Autodesk Inventor part; units mm, degrees
(part 2 of 4)
sketch "スケッチ16" plane through (0, 0, 0) normal (0, 0, 1) x (1, 0, 0)
  line L0 (45.3386, -92.477) -> (54.3014, -95.75) projected
  line L1 (54.3014, -95.75) -> (66.3014, -95.75) projected
  line L2 (66.3014, -95.75) -> (66.3014, -95.339) projected
  arc A0 (74.7167, -80.1031) -> (66.3014, -95.339) centre (84.3014, -95.339) ccw projected
  line L3 (74.7167, -80.1031) -> (119.8722, -51.6966) projected
  arc A1 (119.8722, -51.6966) -> (121.0577, -50.8686) centre (111.885, -39) ccw projected
  line L4 (121.0577, -50.8686) -> (127.6513, -45.7727) projected
  line L5 (127.6513, -45.7727) -> (126.8081, -37.4821) projected
  arc A2 (126.8081, -37.4821) -> (124.1514, -30.3665) centre (111.885, -39) ccw projected
  line L6 (124.1514, -30.3665) -> (104.8897, -3) projected
  line L7 (104.8897, -3) -> (101.8897, -3) projected
  arc A3 (99.8897, -3) -> (101.8897, -3) centre (100.8897, -3) ccw projected
  line L8 (99.8897, -3) -> (99.8897, 0) projected
  line L9 (99.8897, 0) -> (84.8897, 0) projected
  line L10 (84.8897, 0) -> (84.8897, -3) projected
  arc A4 (82.8897, -3) -> (84.8897, -3) centre (83.8897, -3) ccw projected
  line L11 (82.8897, -3) -> (71.4443, -3) projected
  arc A5 (69.4443, -3) -> (71.4443, -3) centre (70.4443, -3) ccw projected
  line L12 (69.4443, -3) -> (69.4443, 0) projected
  line L13 (69.4443, 0) -> (54.4443, 0) projected
  line L14 (54.4443, 0) -> (54.4443, -3) projected
  arc A6 (52.4443, -3) -> (54.4443, -3) centre (53.4443, -3) ccw projected
  line L15 (52.4443, -3) -> (49.4443, -3) projected
  line L16 (49.4443, -3) -> (49.4443, -6) projected
  line L17 (49.4443, -6) -> (53.9457, -9.7931) projected
  arc A7 (54.3014, -10.5578) -> (53.9457, -9.7931) centre (53.3014, -10.5578) ccw projected
  line L18 (54.3014, -10.5578) -> (54.3014, -82.75) projected
  arc A8 (53.3014, -83.75) -> (54.3014, -82.75) centre (53.3014, -82.75) ccw projected
  line L19 (53.3014, -83.75) -> (46.8822, -83.75) projected
  arc A9 (46.8822, -83.75) -> (45.3386, -92.477) centre (46.8822, -88.25) ccw projected
  circle A10 centre (111.885, -39) radius 1.5 projected
  arc A11 (89.8897, -3) -> (87.8897, -3) centre (88.8897, -3) ccw projected
  line L20 (89.8897, -3) -> (94.8897, -3) projected
  arc A12 (96.8897, -3) -> (94.8897, -3) centre (95.8897, -3) ccw projected
  line L21 (96.8897, -3) -> (96.8897, -6) projected
  arc A13 (94.8897, -6) -> (96.8897, -6) centre (95.8897, -6) ccw projected
  line L22 (94.8897, -6) -> (89.8897, -6) projected
  arc A14 (87.8897, -6) -> (89.8897, -6) centre (88.8897, -6) ccw projected
  line L23 (87.8897, -6) -> (87.8897, -3) projected
  line L24 (57.4443, -6) -> (57.4443, -3) projected
  arc A15 (59.4443, -3) -> (57.4443, -3) centre (58.4443, -3) ccw projected
  line L25 (59.4443, -3) -> (64.4443, -3) projected
  arc A16 (66.4443, -3) -> (64.4443, -3) centre (65.4443, -3) ccw projected
  line L26 (66.4443, -3) -> (66.4443, -6) projected
  arc A17 (64.4443, -6) -> (66.4443, -6) centre (65.4443, -6) ccw projected
  line L27 (64.4443, -6) -> (59.4443, -6) projected
  arc A18 (57.4443, -6) -> (59.4443, -6) centre (58.4443, -6) ccw projected
  circle A19 centre (46.8822, -88.25) radius 1.5 projected
  circle A20 centre (47.8869, -88.25) radius 1.5
  line L28 (46.177, -92.4125) -> (54.3014, -95.75)
  line L29 (54.3014, -95.75) -> (66.3014, -95.75)
  line L30 (66.3014, -95.75) -> (66.3014, -95.339)
  arc A21 (74.7167, -80.1031) -> (66.3014, -95.339) centre (84.3014, -95.339) ccw
  line L31 (74.7167, -80.1031) -> (119.8722, -51.6966)
  arc A22 (119.8722, -51.6966) -> (121.0577, -50.8686) centre (111.885, -39) ccw
  line L32 (121.0577, -50.8686) -> (127.6513, -45.7727)
  line L33 (127.6513, -45.7727) -> (119.127, -45.896)
  arc A23 (104.885, -31.8586) -> (119.127, -45.896) centre (111.885, -39) ccw
  line L34 (104.885, -31.8586) -> (104.885, -3)
  line L35 (104.885, -3) -> (101.8897, -3)
  arc A24 (99.8897, -3) -> (101.8897, -3) centre (100.8897, -3) ccw
  line L36 (99.8897, -3) -> (96.8897, -3)
  line L37 (96.8897, -3) -> (96.8897, -6)
  arc A25 (94.8897, -6) -> (96.8897, -6) centre (95.8897, -6) ccw
  line L38 (94.8897, -6) -> (89.8897, -6)
  arc A26 (87.8897, -6) -> (89.8897, -6) centre (88.8897, -6) ccw
  line L39 (87.8897, -6) -> (87.8897, -3)
  line L40 (87.8897, -3) -> (84.8897, -3)
  arc A27 (82.8897, -3) -> (84.8897, -3) centre (83.8897, -3) ccw
  line L41 (82.8897, -3) -> (71.4443, -3)
  arc A28 (69.4443, -3) -> (71.4443, -3) centre (70.4443, -3) ccw
  line L42 (69.4443, -3) -> (66.4443, -3)
  line L43 (66.4443, -3) -> (66.4443, -6)
  arc A29 (64.4443, -6) -> (66.4443, -6) centre (65.4443, -6) ccw
  line L44 (64.4443, -6) -> (59.4443, -6)
  arc A30 (57.4443, -6) -> (59.4443, -6) centre (58.4443, -6) ccw
  line L45 (57.4443, -6) -> (57.4443, -3)
  line L46 (57.4443, -3) -> (54.4443, -3)
  arc A31 (52.4443, -3) -> (54.4443, -3) centre (53.4443, -3) ccw
  line L47 (52.4443, -3) -> (49.4443, -3)
  line L48 (49.4443, -3) -> (49.4443, -6)
  line L49 (49.4443, -6) -> (53.9457, -9.7931)
  arc A32 (54.3014, -10.5578) -> (53.9457, -9.7931) centre (53.3014, -10.5578) ccw
  line L50 (54.3014, -10.5578) -> (54.3014, -82.75)
  arc A33 (53.3014, -83.75) -> (54.3014, -82.75) centre (53.3014, -82.75) ccw
  line L51 (53.3014, -83.75) -> (47.8869, -83.75)
  arc A34 (47.8869, -83.75) -> (46.177, -92.4125) centre (47.8869, -88.25) ccw
  point P0 (0, 0)
  point P1 (0, 0)
  point P2 (47.885, -83.75)
  constraints: 48 end point, 28 point on circle, 21 horizontal, 19 vertical, 15 centre point, 168 other
extrude "押し出し19" add sketch "スケッチ16" against normal blind 5 contours A19 A20 | A20 A19 picked at (47.067, -88.3717) picked at (46.0813, -88.0099)
extrude "押し出し20" cut sketch "スケッチ16" against normal blind 10 contours A9 L19 A34 L28 L0
hole "穴2" at (47.8869, -88.25, 0) direction (0, 0, -1) diameter 3 depth 12 tip angle 118
sketch "スケッチ17" plane through (0, 0, -5) normal (0, 0, -1) x (-1, 0, 0)
  circle A0 centre (-47.8869, -88.25) radius 1.5 projected
  arc A1 (-46.177, -92.4125) -> (-47.885, -83.75) centre (-47.8869, -88.25) ccw projected
  line L0 (-47.885, -83.75) -> (-53.3014, -83.75) projected
  arc A2 (-54.3014, -82.75) -> (-53.3014, -83.75) centre (-53.3014, -82.75) ccw projected
  line L1 (-54.3014, -82.75) -> (-54.3014, -10.5578) projected
  arc A3 (-53.9457, -9.7931) -> (-54.3014, -10.5578) centre (-53.3014, -10.5578) ccw projected
  line L2 (-53.9457, -9.7931) -> (-49.4443, -6) projected
  line L3 (-49.4443, -6) -> (-49.4443, -3) projected
  line L4 (-49.4443, -3) -> (-52.4443, -3) projected
  arc A4 (-54.4443, -3) -> (-52.4443, -3) centre (-53.4443, -3) ccw projected
  line L5 (-54.4443, -3) -> (-57.4443, -3) projected
  line L6 (-57.4443, -3) -> (-57.4443, -6) projected
  arc A5 (-59.4443, -6) -> (-57.4443, -6) centre (-58.4443, -6) ccw projected
  line L7 (-59.4443, -6) -> (-64.4443, -6) projected
  arc A6 (-66.4443, -6) -> (-64.4443, -6) centre (-65.4443, -6) ccw projected
  line L8 (-66.4443, -6) -> (-66.4443, -3) projected
  line L9 (-66.4443, -3) -> (-69.4443, -3) projected
  arc A7 (-71.4443, -3) -> (-69.4443, -3) centre (-70.4443, -3) ccw projected
  line L10 (-71.4443, -3) -> (-82.8897, -3) projected
  arc A8 (-84.8897, -3) -> (-82.8897, -3) centre (-83.8897, -3) ccw projected
  line L11 (-84.8897, -3) -> (-87.8897, -3) projected
  line L12 (-87.8897, -3) -> (-87.8897, -6) projected
  arc A9 (-89.8897, -6) -> (-87.8897, -6) centre (-88.8897, -6) ccw projected
  line L13 (-89.8897, -6) -> (-94.8897, -6) projected
  arc A10 (-96.8897, -6) -> (-94.8897, -6) centre (-95.8897, -6) ccw projected
  line L14 (-96.8897, -6) -> (-96.8897, -3) projected
  line L15 (-96.8897, -3) -> (-99.8897, -3) projected
  arc A11 (-101.8897, -3) -> (-99.8897, -3) centre (-100.8897, -3) ccw projected
  line L16 (-101.8897, -3) -> (-104.885, -3) projected
  line L17 (-104.885, -3) -> (-104.885, -31.8586) projected
  arc A12 (-119.127, -45.896) -> (-104.885, -31.8586) centre (-111.885, -39) ccw projected
  line L18 (-119.127, -45.896) -> (-127.6513, -45.7727) projected
  line L19 (-127.6513, -45.7727) -> (-121.0577, -50.8686) projected
  arc A13 (-121.0577, -50.8686) -> (-119.8722, -51.6966) centre (-111.885, -39) ccw projected
  line L20 (-119.8722, -51.6966) -> (-74.7167, -80.1031) projected
  arc A14 (-66.3014, -95.339) -> (-74.7167, -80.1031) centre (-84.3014, -95.339) ccw projected
  line L21 (-66.3014, -95.339) -> (-66.3014, -95.75) projected
  line L22 (-66.3014, -95.75) -> (-54.3014, -95.75) projected
  line L23 (-54.3014, -95.75) -> (-46.177, -92.4125) projected
  line L24 (-71.5218, -75.0244) -> (-116.6774, -46.618)
  arc A15 (-117.3886, -46.1211) -> (-116.6774, -46.618) centre (-111.885, -39) ccw
  line L25 (-117.3886, -46.1211) -> (-127.8557, -38.0317)
  arc A16 (-127.8557, -38.0317) -> (-98.885, -29.6726) centre (-111.885, -39) ccw
  line L26 (-98.885, -29.6726) -> (-98.885, -12.3268)
  arc A17 (-98.885, -12.3268) -> (-92.3897, -12.0622) centre (-95.8897, -6) ccw
  arc A18 (-92.3897, -12.0622) -> (-81.8897, -6) centre (-88.8897, -6) ccw
  line L27 (-81.8897, -6) -> (-81.8897, 3.7082)
  arc A19 (-81.8897, 3.7082) -> (-80.2841, -9) centre (-83.8897, -3) ccw
  line L28 (-80.2841, -9) -> (-74.0499, -9)
  arc A20 (-74.0499, -9) -> (-72.4443, 3.7082) centre (-70.4443, -3) ccw
  line L29 (-72.4443, 3.7082) -> (-72.4443, -6)
  arc A21 (-72.4443, -6) -> (-61.9443, 0.0622) centre (-65.4443, -6) ccw
  arc A22 (-61.9443, 0.0622) -> (-60.3014, -12.7492) centre (-58.4443, -6) ccw
  line L30 (-60.3014, -12.7492) -> (-60.3014, -82.75)
  arc A23 (-60.3014, -82.75) -> (-54.9853, -89.5444) centre (-53.3014, -82.75) ccw
  line L31 (-54.9853, -89.5444) -> (-55.4858, -89.75)
  line L32 (-55.4858, -89.75) -> (-60.9612, -89.75)
  arc A24 (-60.9612, -89.75) -> (-71.5218, -75.0244) centre (-84.3014, -95.339) ccw
  arc A25 (-58.5929, -89.75) -> (-57.9314, -88) centre (-58.5929, -88.75) ccw
  point P0 (0, 0)
  point P1 (-105.48, -53.662)
  point P2 (-61.9443, -12.0622)
  point P3 (-71.2186, -9.9571)
  point P4 (-83.1155, -9.9571)
  dimension "d164" = 6
  dimension "d166" = 2
  constraints: 23 point on circle, 18 end point, 11 centre point, 2 tangent, 1 point on line, 18 other
  measures "d164" distance between parallel lines of L20 L24
  measures "d166" diameter of A25
extrude "押し出し21" cut sketch "スケッチ17" against normal blind 4 contours A16 L26 A17 A18 A19 L28 A20 A21 A22 L30 A23 A25 L32 A24 L24
fillet "フィレット3" radius 1 11 edges at (60.9612, -89.75, -3) (105.48, -53.662, -3) (98.885, -29.6726, -3) (98.885, -12.3268, -3) (92.3897, -12.0622, -3) (83.1155, -9.9571, -3) (80.2841, -9, -3) (74.0499, -9, -3) (71.2186, -9.9571, -3) (61.9443, -12.0622, -3) (60.3014, -12.7492, -3)
sketch "スケッチ18" plane through (0, 0, -5) normal (0, 0, -1) x (-1, 0, 0)
  arc A0 (-82.7234, -9.9022) -> (-80.5008, -9.125) centre (-83.8897, -3) ccw projected
  arc A1 (-80.0167, -9) -> (-80.5008, -9.125) centre (-80.0167, -10) ccw projected
  line L0 (-80.0167, -9) -> (-74.3173, -9) projected
  arc A2 (-73.8332, -9.125) -> (-74.3173, -9) centre (-74.3173, -10) ccw projected
  arc A3 (-73.8332, -9.125) -> (-71.6106, -9.9022) centre (-70.4443, -3) ccw projected
  arc A4 (-70.9856, -10.2772) -> (-71.6106, -9.9022) centre (-71.7772, -10.8882) ccw projected
  arc A5 (-70.9856, -10.2772) -> (-62.3818, -12.2945) centre (-65.4443, -6) ccw projected
  arc A6 (-61.5068, -12.2945) -> (-62.3818, -12.2945) centre (-61.9443, -13.1937) ccw projected
  arc A7 (-61.5068, -12.2945) -> (-60.9442, -12.5384) centre (-58.4443, -6) ccw projected
  arc A8 (-60.3014, -13.4724) -> (-60.9442, -12.5384) centre (-61.3014, -13.4724) ccw projected
  line L1 (-60.3014, -13.4724) -> (-60.3014, -82.75) projected
  arc A9 (-60.3014, -82.75) -> (-57.9314, -88) centre (-53.3014, -82.75) ccw projected
  arc A10 (-58.5929, -89.75) -> (-57.9314, -88) centre (-58.5929, -88.75) ccw projected
  line L2 (-58.5929, -89.75) -> (-60.1853, -89.75) projected
  arc A11 (-61.1499, -89.0136) -> (-60.1853, -89.75) centre (-60.1853, -88.75) ccw projected
  arc A12 (-61.1499, -89.0136) -> (-71.5218, -75.0244) centre (-84.3014, -95.339) ccw projected
  line L3 (-71.5218, -75.0244) -> (-103.9807, -54.6052) projected
  arc A13 (-103.9445, -52.8906) -> (-103.9807, -54.6052) centre (-103.4483, -53.7587) ccw projected
  arc A14 (-103.9445, -52.8906) -> (-98.7086, -29.9236) centre (-111.885, -39) ccw projected
  arc A15 (-98.885, -29.3564) -> (-98.7086, -29.9236) centre (-97.885, -29.3564) ccw projected
  line L4 (-98.885, -29.3564) -> (-98.885, -13.7472) projected
  arc A16 (-97.6356, -12.7788) -> (-98.885, -13.7472) centre (-97.885, -13.7472) ccw projected
  arc A17 (-97.6356, -12.7788) -> (-92.8272, -12.2945) centre (-95.8897, -6) ccw projected
  arc A18 (-91.9522, -12.2945) -> (-92.8272, -12.2945) centre (-92.3897, -13.1937) ccw projected
  arc A19 (-91.9522, -12.2945) -> (-83.3484, -10.2772) centre (-88.8897, -6) ccw projected
  arc A20 (-82.7234, -9.9022) -> (-83.3484, -10.2772) centre (-82.5568, -10.8882) ccw projected
  circle A21 centre (-47.8869, -88.25) radius 1.5 projected
  arc A22 (-46.177, -92.4125) -> (-47.885, -83.75) centre (-47.8869, -88.25) ccw projected
  line L5 (-47.885, -83.75) -> (-53.3014, -83.75) projected
  arc A23 (-54.3014, -82.75) -> (-53.3014, -83.75) centre (-53.3014, -82.75) ccw projected
  line L6 (-54.3014, -82.75) -> (-54.3014, -10.5578) projected
  arc A24 (-53.9457, -9.7931) -> (-54.3014, -10.5578) centre (-53.3014, -10.5578) ccw projected
  line L7 (-53.9457, -9.7931) -> (-49.4443, -6) projected
  line L8 (-49.4443, -6) -> (-49.4443, -3) projected
  line L9 (-49.4443, -3) -> (-52.4443, -3) projected
  arc A25 (-54.4443, -3) -> (-52.4443, -3) centre (-53.4443, -3) ccw projected
  line L10 (-54.4443, -3) -> (-57.4443, -3) projected
  line L11 (-57.4443, -3) -> (-57.4443, -6) projected
  arc A26 (-59.4443, -6) -> (-57.4443, -6) centre (-58.4443, -6) ccw projected
  line L12 (-59.4443, -6) -> (-64.4443, -6) projected
  arc A27 (-66.4443, -6) -> (-64.4443, -6) centre (-65.4443, -6) ccw projected
  line L13 (-66.4443, -6) -> (-66.4443, -3) projected
  line L14 (-66.4443, -3) -> (-69.4443, -3) projected
  arc A28 (-71.4443, -3) -> (-69.4443, -3) centre (-70.4443, -3) ccw projected
  line L15 (-71.4443, -3) -> (-82.8897, -3) projected
  arc A29 (-84.8897, -3) -> (-82.8897, -3) centre (-83.8897, -3) ccw projected
  line L16 (-84.8897, -3) -> (-87.8897, -3) projected
  line L17 (-87.8897, -3) -> (-87.8897, -6) projected
  arc A30 (-89.8897, -6) -> (-87.8897, -6) centre (-88.8897, -6) ccw projected
  line L18 (-89.8897, -6) -> (-94.8897, -6) projected
  arc A31 (-96.8897, -6) -> (-94.8897, -6) centre (-95.8897, -6) ccw projected
  line L19 (-96.8897, -6) -> (-96.8897, -3) projected
  line L20 (-96.8897, -3) -> (-99.8897, -3) projected
  arc A32 (-101.8897, -3) -> (-99.8897, -3) centre (-100.8897, -3) ccw projected
  line L21 (-101.8897, -3) -> (-104.885, -3) projected
  line L22 (-104.885, -3) -> (-104.885, -31.8586) projected
  arc A33 (-119.127, -45.896) -> (-104.885, -31.8586) centre (-111.885, -39) ccw projected
  line L23 (-119.127, -45.896) -> (-127.6513, -45.7727) projected
  line L24 (-127.6513, -45.7727) -> (-121.0577, -50.8686) projected
  arc A34 (-121.0577, -50.8686) -> (-119.8722, -51.6966) centre (-111.885, -39) ccw projected
  line L25 (-119.8722, -51.6966) -> (-74.7167, -80.1031) projected
  arc A35 (-66.3014, -95.339) -> (-74.7167, -80.1031) centre (-84.3014, -95.339) ccw projected
  line L26 (-66.3014, -95.339) -> (-66.3014, -95.75) projected
  line L27 (-66.3014, -95.75) -> (-54.3014, -95.75) projected
  line L28 (-54.3014, -95.75) -> (-46.177, -92.4125) projected
  line L29 (-105.5782, -57.1445) -> (-73.1193, -77.5638)
  arc A36 (-64.0439, -89.8042) -> (-73.1193, -77.5638) centre (-84.3014, -95.339) ccw
  arc A37 (-64.0439, -89.8042) -> (-60.1853, -92.75) centre (-60.1853, -88.75) ccw
  line L30 (-60.1853, -92.75) -> (-58.5929, -92.75)
  arc A38 (-58.5929, -92.75) -> (-55.9471, -85.75) centre (-58.5929, -88.75) ccw
  arc A39 (-57.3014, -82.75) -> (-55.9471, -85.75) centre (-53.3014, -82.75) ccw
  line L31 (-57.3014, -82.75) -> (-57.3014, -13.4724)
  arc A40 (-57.3014, -13.4724) -> (-59.8728, -9.7362) centre (-61.3014, -13.4724) ccw
  arc A41 (-60.1943, -9.5969) -> (-59.8728, -9.7362) centre (-58.4443, -6) ccw
  arc A42 (-60.1943, -9.5969) -> (-63.6943, -9.5969) centre (-61.9443, -13.1937) ccw
  arc A43 (-68.6108, -8.4441) -> (-63.6943, -9.5969) centre (-65.4443, -6) ccw
  arc A44 (-68.6108, -8.4441) -> (-71.1108, -6.9441) centre (-71.7772, -10.8882) ccw
  arc A45 (-72.3808, -6.5) -> (-71.1108, -6.9441) centre (-70.4443, -3) ccw
  arc A46 (-72.3808, -6.5) -> (-74.3173, -6) centre (-74.3173, -10) ccw
  line L32 (-74.3173, -6) -> (-80.0167, -6)
  arc A47 (-80.0167, -6) -> (-81.9532, -6.5) centre (-80.0167, -10) ccw
  arc A48 (-83.2232, -6.9441) -> (-81.9532, -6.5) centre (-83.8897, -3) ccw
  arc A49 (-83.2232, -6.9441) -> (-85.7232, -8.4441) centre (-82.5568, -10.8882) ccw
  arc A50 (-90.6397, -9.5969) -> (-85.7232, -8.4441) centre (-88.8897, -6) ccw
  arc A51 (-90.6397, -9.5969) -> (-94.1397, -9.5969) centre (-92.3897, -13.1937) ccw
  arc A52 (-96.8874, -9.8736) -> (-94.1397, -9.5969) centre (-95.8897, -6) ccw
  arc A53 (-96.8874, -9.8736) -> (-101.885, -13.7472) centre (-97.885, -13.7472) ccw
  line L33 (-101.885, -13.7472) -> (-101.885, -29.3564)
  arc A54 (-101.885, -29.3564) -> (-101.1792, -31.6254) centre (-97.885, -29.3564) ccw
  arc A55 (-105.4334, -50.2861) -> (-101.1792, -31.6254) centre (-111.885, -39) ccw
  arc A56 (-105.4334, -50.2861) -> (-105.5782, -57.1445) centre (-103.4483, -53.7587) ccw
  arc A57 (-103.9445, -52.8906) -> (-98.7086, -29.9236) centre (-111.885, -39) ccw projected
  line L34 (-100.6732, -50.4147) -> (-60.5392, -10.9939)
  arc A58 (-103.9445, -52.8906) -> (-98.7086, -29.9236) centre (-111.885, -39) ccw projected
  arc A59 (-70.9856, -10.2772) -> (-62.3818, -12.2945) centre (-65.4443, -6) ccw projected
  line L35 (-104.8777, -46.1342) -> (-64.7436, -6.7134)
  point P0 (0, 0)
  dimension "d171" = 3
  dimension "d172" = 6
  constraints: 44 point on circle, 21 centre point, 14 end point, 2 tangent, 1 parallel, 25 other
  measures "d171" distance between parallel lines of L3 L29
  measures "d172" distance between parallel lines of L34 L35
sketch "スケッチ19" plane through (0, 0, -5) normal (0, 0, -1) x (-1, 0, 0)
  line L0 (-98.885, -17.6269) -> (-98.885, -29.3564)
  arc A0 (-98.885, -29.3564) -> (-98.7086, -29.9236) centre (-97.885, -29.3564) ccw
  arc A1 (-96.2374, -35.6607) -> (-98.7086, -29.9236) centre (-111.885, -39) ccw
  arc A2 (-96.2374, -35.6607) -> (-94.615, -36.2167) centre (-95.2594, -35.452) ccw
  line L1 (-94.615, -36.2167) -> (-87.3669, -30.1091)
  arc A3 (-87.3669, -30.1091) -> (-87.2466, -28.7001) centre (-88.0113, -29.3444) ccw
  line L2 (-87.2466, -28.7001) -> (-97.1203, -16.9825)
  arc A4 (-97.1203, -16.9825) -> (-98.885, -17.6269) centre (-97.885, -17.6269) ccw
  line L3 (-95.2693, -14.5236) -> (-84.9525, -26.7669)
  arc A5 (-84.9525, -26.7669) -> (-83.5434, -26.8873) centre (-84.1878, -26.1225) ccw
  line L4 (-83.5434, -26.8873) -> (-68.2365, -13.989)
  arc A6 (-68.2365, -13.989) -> (-68.4513, -12.3212) centre (-68.8809, -13.2243) ccw
  arc A7 (-70.9856, -10.2772) -> (-68.4513, -12.3212) centre (-65.4443, -6) ccw
  arc A8 (-70.9856, -10.2772) -> (-71.6106, -9.9022) centre (-71.7772, -10.8882) ccw
  arc A9 (-73.8332, -9.125) -> (-71.6106, -9.9022) centre (-70.4443, -3) ccw
  arc A10 (-73.8332, -9.125) -> (-74.3173, -9) centre (-74.3173, -10) ccw
  line L5 (-74.3173, -9) -> (-80.0167, -9)
  arc A11 (-80.0167, -9) -> (-80.5008, -9.125) centre (-80.0167, -10) ccw
  arc A12 (-82.7234, -9.9022) -> (-80.5008, -9.125) centre (-83.8897, -3) ccw
  arc A13 (-82.7234, -9.9022) -> (-83.3484, -10.2772) centre (-82.5568, -10.8882) ccw
  arc A14 (-91.9522, -12.2945) -> (-83.3484, -10.2772) centre (-88.8897, -6) ccw
  arc A15 (-91.9522, -12.2945) -> (-92.8272, -12.2945) centre (-92.3897, -13.1937) ccw
  arc A16 (-94.6777, -12.8943) -> (-92.8272, -12.2945) centre (-95.8897, -6) ccw
  arc A17 (-94.6777, -12.8943) -> (-95.2693, -14.5236) centre (-94.5046, -13.8792) ccw
  line L6 (-57.4443, -3) -> (-54.4443, -3)
  arc A18 (-54.4443, -3) -> (-52.4443, -3) centre (-53.4443, -3) ccw
  line L7 (-52.4443, -3) -> (-49.4443, -3)
  line L8 (-49.4443, -3) -> (-49.4443, -6)
  line L9 (-49.4443, -6) -> (-102.2194, -50.4706)
  arc A19 (-121.0577, -50.8686) -> (-102.2194, -50.4706) centre (-111.885, -39) ccw
  line L10 (-121.0577, -50.8686) -> (-127.6513, -45.7727)
  line L11 (-127.6513, -45.7727) -> (-119.127, -45.896)
  arc A20 (-119.127, -45.896) -> (-104.885, -31.8586) centre (-111.885, -39) ccw
  line L12 (-104.885, -31.8586) -> (-104.885, -3)
  line L13 (-104.885, -3) -> (-101.8897, -3)
  arc A21 (-101.8897, -3) -> (-99.8897, -3) centre (-100.8897, -3) ccw
  line L14 (-99.8897, -3) -> (-96.8897, -3)
  line L15 (-96.8897, -3) -> (-96.8897, -6)
  arc A22 (-96.8897, -6) -> (-94.8897, -6) centre (-95.8897, -6) ccw
  line L16 (-94.8897, -6) -> (-89.8897, -6)
  arc A23 (-89.8897, -6) -> (-87.8897, -6) centre (-88.8897, -6) ccw
  line L17 (-87.8897, -6) -> (-87.8897, -3)
  line L18 (-87.8897, -3) -> (-84.8897, -3)
  arc A24 (-84.8897, -3) -> (-82.8897, -3) centre (-83.8897, -3) ccw
  line L19 (-82.8897, -3) -> (-71.4443, -3)
  arc A25 (-71.4443, -3) -> (-69.4443, -3) centre (-70.4443, -3) ccw
  line L20 (-69.4443, -3) -> (-66.4443, -3)
  line L21 (-66.4443, -3) -> (-66.4443, -6)
  arc A26 (-66.4443, -6) -> (-64.4443, -6) centre (-65.4443, -6) ccw
  line L22 (-64.4443, -6) -> (-59.4443, -6)
  arc A27 (-59.4443, -6) -> (-57.4443, -6) centre (-58.4443, -6) ccw
  line L23 (-57.4443, -6) -> (-57.4443, -3)
  line L24 (-107.885, -23.7831) -> (-107.885, -15.6261)
  arc A28 (-107.885, -15.6261) -> (-109.7028, -15.0506) centre (-108.885, -15.6261) ccw
  line L25 (-109.7028, -15.0506) -> (-113.5421, -20.5053)
  arc A29 (-113.5421, -20.5053) -> (-113.2999, -21.8986) centre (-112.7243, -21.0809) ccw
  line L26 (-113.2999, -21.8986) -> (-109.4606, -24.6009)
  arc A30 (-109.4606, -24.6009) -> (-107.885, -23.7831) centre (-108.885, -23.7831) ccw
  arc A31 (-123.011, -34.5042) -> (-123.8235, -37.7857) centre (-111.885, -39) ccw
  line L27 (-123.8235, -37.7857) -> (-124.2252, -41.735)
  arc A32 (-124.2252, -41.735) -> (-123.2447, -42.8361) centre (-123.2303, -41.8362) ccw
  line L28 (-123.2447, -42.8361) -> (-120.4273, -42.8769)
  arc A33 (-120.4273, -42.8769) -> (-119.4653, -41.5573) centre (-120.4128, -41.877) ccw
  arc A34 (-119.4487, -36.3939) -> (-119.4653, -41.5573) centre (-111.885, -39) ccw
  arc A35 (-119.4487, -36.3939) -> (-119.8185, -35.2504) centre (-120.3941, -36.0681) ccw
  line L29 (-119.8185, -35.2504) -> (-121.5083, -34.0611)
  arc A36 (-121.5083, -34.0611) -> (-123.011, -34.5042) centre (-122.0839, -34.8788) ccw
  line L30 (-108.3095, -29.0797) -> (-115.0266, -24.3519)
  arc A37 (-115.0266, -24.3519) -> (-116.4199, -24.5941) centre (-115.6022, -25.1696) ccw
  line L31 (-116.4199, -24.5941) -> (-120.2592, -30.0488)
  arc A38 (-120.2592, -30.0488) -> (-120.017, -31.4421) centre (-119.4414, -30.6244) ccw
  line L32 (-120.017, -31.4421) -> (-118.0918, -32.7971)
  arc A39 (-118.0918, -32.7971) -> (-116.8906, -32.7594) centre (-117.5163, -31.9794) ccw
  arc A40 (-109.2184, -31.4575) -> (-116.8906, -32.7594) centre (-111.885, -39) ccw
  arc A41 (-109.2184, -31.4575) -> (-107.885, -30.5147) centre (-108.885, -30.5147) ccw
  line L33 (-107.885, -30.5147) -> (-107.885, -29.8974)
  arc A42 (-107.885, -29.8974) -> (-108.3095, -29.0797) centre (-108.885, -29.8974) ccw
  circle A43 centre (-111.885, -39) radius 3
  line L34 (-104.885, -3) -> (-104.8897, -3)
  line L35 (-104.885, -31.8586) -> (-104.885, -3)
  arc A44 (-119.127, -45.896) -> (-104.885, -31.8586) centre (-111.885, -39) ccw
  line L36 (-127.6513, -45.7727) -> (-119.127, -45.896)
  line L37 (-126.8081, -37.4821) -> (-127.6513, -45.7727)
  arc A45 (-124.1514, -30.3665) -> (-126.8081, -37.4821) centre (-111.885, -39) ccw
  line L38 (-104.8897, -3) -> (-124.1514, -30.3665)
  arc A46 (-82.7234, -9.9022) -> (-80.5008, -9.125) centre (-83.8897, -3) ccw projected
  arc A47 (-80.0167, -9) -> (-80.5008, -9.125) centre (-80.0167, -10) ccw projected
  line L39 (-80.0167, -9) -> (-74.3173, -9) projected
  arc A48 (-73.8332, -9.125) -> (-74.3173, -9) centre (-74.3173, -10) ccw projected
  arc A49 (-73.8332, -9.125) -> (-71.6106, -9.9022) centre (-70.4443, -3) ccw projected
  arc A50 (-70.9856, -10.2772) -> (-71.6106, -9.9022) centre (-71.7772, -10.8882) ccw projected
  arc A51 (-70.9856, -10.2772) -> (-62.3818, -12.2945) centre (-65.4443, -6) ccw projected
  arc A52 (-61.5068, -12.2945) -> (-62.3818, -12.2945) centre (-61.9443, -13.1937) ccw projected
  arc A53 (-61.5068, -12.2945) -> (-60.9442, -12.5384) centre (-58.4443, -6) ccw projected
  arc A54 (-60.3014, -13.4724) -> (-60.9442, -12.5384) centre (-61.3014, -13.4724) ccw projected
  line L40 (-60.3014, -13.4724) -> (-60.3014, -82.75) projected
  arc A55 (-60.3014, -82.75) -> (-57.9314, -88) centre (-53.3014, -82.75) ccw projected
  arc A56 (-58.5929, -89.75) -> (-57.9314, -88) centre (-58.5929, -88.75) ccw projected
  line L41 (-58.5929, -89.75) -> (-60.1853, -89.75) projected
  arc A57 (-61.1499, -89.0136) -> (-60.1853, -89.75) centre (-60.1853, -88.75) ccw projected
  arc A58 (-61.1499, -89.0136) -> (-71.5218, -75.0244) centre (-84.3014, -95.339) ccw projected
  line L42 (-71.5218, -75.0244) -> (-103.9807, -54.6052) projected
  arc A59 (-103.9445, -52.8906) -> (-103.9807, -54.6052) centre (-103.4483, -53.7587) ccw projected
  arc A60 (-103.9445, -52.8906) -> (-98.7086, -29.9236) centre (-111.885, -39) ccw projected
  arc A61 (-98.885, -29.3564) -> (-98.7086, -29.9236) centre (-97.885, -29.3564) ccw projected
  line L43 (-98.885, -29.3564) -> (-98.885, -13.7472) projected
  arc A62 (-97.6356, -12.7788) -> (-98.885, -13.7472) centre (-97.885, -13.7472) ccw projected
  arc A63 (-97.6356, -12.7788) -> (-92.8272, -12.2945) centre (-95.8897, -6) ccw projected
  arc A64 (-91.9522, -12.2945) -> (-92.8272, -12.2945) centre (-92.3897, -13.1937) ccw projected
  arc A65 (-91.9522, -12.2945) -> (-83.3484, -10.2772) centre (-88.8897, -6) ccw projected
  arc A66 (-82.7234, -9.9022) -> (-83.3484, -10.2772) centre (-82.5568, -10.8882) ccw projected
  circle A67 centre (-47.8869, -88.25) radius 1.5 projected
  arc A68 (-46.177, -92.4125) -> (-47.885, -83.75) centre (-47.8869, -88.25) ccw projected
  line L44 (-47.885, -83.75) -> (-53.3014, -83.75) projected
  arc A69 (-54.3014, -82.75) -> (-53.3014, -83.75) centre (-53.3014, -82.75) ccw projected
  line L45 (-54.3014, -82.75) -> (-54.3014, -10.5578) projected
  arc A70 (-53.9457, -9.7931) -> (-54.3014, -10.5578) centre (-53.3014, -10.5578) ccw projected
  line L46 (-53.9457, -9.7931) -> (-49.4443, -6) projected
  line L47 (-49.4443, -6) -> (-49.4443, -3) projected
  line L48 (-49.4443, -3) -> (-52.4443, -3) projected
  arc A71 (-54.4443, -3) -> (-52.4443, -3) centre (-53.4443, -3) ccw projected
  line L49 (-54.4443, -3) -> (-57.4443, -3) projected
  line L50 (-57.4443, -3) -> (-57.4443, -6) projected
  arc A72 (-59.4443, -6) -> (-57.4443, -6) centre (-58.4443, -6) ccw projected
  line L51 (-59.4443, -6) -> (-64.4443, -6) projected
  arc A73 (-66.4443, -6) -> (-64.4443, -6) centre (-65.4443, -6) ccw projected
  line L52 (-66.4443, -6) -> (-66.4443, -3) projected
  line L53 (-66.4443, -3) -> (-69.4443, -3) projected
  arc A74 (-71.4443, -3) -> (-69.4443, -3) centre (-70.4443, -3) ccw projected
  line L54 (-71.4443, -3) -> (-82.8897, -3) projected
  arc A75 (-84.8897, -3) -> (-82.8897, -3) centre (-83.8897, -3) ccw projected
  line L55 (-84.8897, -3) -> (-87.8897, -3) projected
  line L56 (-87.8897, -3) -> (-87.8897, -6) projected
  arc A76 (-89.8897, -6) -> (-87.8897, -6) centre (-88.8897, -6) ccw projected
  line L57 (-89.8897, -6) -> (-94.8897, -6) projected
  arc A77 (-96.8897, -6) -> (-94.8897, -6) centre (-95.8897, -6) ccw projected
  line L58 (-96.8897, -6) -> (-96.8897, -3) projected
  line L59 (-96.8897, -3) -> (-99.8897, -3) projected
  arc A78 (-101.8897, -3) -> (-99.8897, -3) centre (-100.8897, -3) ccw projected
  line L60 (-101.8897, -3) -> (-104.885, -3) projected
  line L61 (-104.885, -3) -> (-104.885, -31.8586) projected
  arc A79 (-119.127, -45.896) -> (-104.885, -31.8586) centre (-111.885, -39) ccw projected
  line L62 (-119.127, -45.896) -> (-127.6513, -45.7727) projected
  line L63 (-127.6513, -45.7727) -> (-121.0577, -50.8686) projected
  arc A80 (-121.0577, -50.8686) -> (-119.8722, -51.6966) centre (-111.885, -39) ccw projected
  line L64 (-119.8722, -51.6966) -> (-74.7167, -80.1031) projected
  arc A81 (-66.3014, -95.339) -> (-74.7167, -80.1031) centre (-84.3014, -95.339) ccw projected
  line L65 (-66.3014, -95.339) -> (-66.3014, -95.75) projected
  line L66 (-66.3014, -95.75) -> (-54.3014, -95.75) projected
  line L67 (-54.3014, -95.75) -> (-46.177, -92.4125) projected
  point P0 (0, 0)
  point P1 (0, 0)
  point P2 (-97.9617, -46.8829)
  point P3 (-60.3014, -15.1486)
  point P4 (-68.4513, -12.3212)
  point P5 (-94.6777, -12.8943)
  constraints: 90 point on circle, 78 end point, 46 centre point, 11 horizontal, 10 vertical, 196 other
extrude "押し出し22" add sketch "スケッチ19" against normal blind 5 contours L43 A62 A63 A17 L3 A5 L4 A6 A51 A52 A53 A54 L40 L9 A60 A2 L1 A3 L2 A4
fillet "フィレット4" radius 1 2 edges at (60.3014, -15.1486, -3) (97.9617, -46.8829, -3)
sketch "スケッチ20" plane through (0, 0, -5) normal (0, 0, -1) x (-1, 0, 0)
  arc A0 (-94.6777, -12.8943) -> (-92.8272, -12.2945) centre (-95.8897, -6) ccw projected
  arc A1 (-91.9522, -12.2945) -> (-92.8272, -12.2945) centre (-92.3897, -13.1937) ccw projected
  arc A2 (-91.9522, -12.2945) -> (-83.3484, -10.2772) centre (-88.8897, -6) ccw projected
  arc A3 (-82.7234, -9.9022) -> (-83.3484, -10.2772) centre (-82.5568, -10.8882) ccw projected
  arc A4 (-82.7234, -9.9022) -> (-80.5008, -9.125) centre (-83.8897, -3) ccw projected
  arc A5 (-80.0167, -9) -> (-80.5008, -9.125) centre (-80.0167, -10) ccw projected
  line L0 (-80.0167, -9) -> (-74.3173, -9) projected
  arc A6 (-73.8332, -9.125) -> (-74.3173, -9) centre (-74.3173, -10) ccw projected
  arc A7 (-73.8332, -9.125) -> (-71.6106, -9.9022) centre (-70.4443, -3) ccw projected
  arc A8 (-70.9856, -10.2772) -> (-71.6106, -9.9022) centre (-71.7772, -10.8882) ccw projected
  arc A9 (-70.9856, -10.2772) -> (-68.4513, -12.3212) centre (-65.4443, -6) ccw projected
  arc A10 (-68.2365, -13.989) -> (-68.4513, -12.3212) centre (-68.8809, -13.2243) ccw projected
  line L1 (-68.2365, -13.989) -> (-83.5434, -26.8873) projected
  arc A11 (-84.9525, -26.7669) -> (-83.5434, -26.8873) centre (-84.1878, -26.1225) ccw projected
  line L2 (-84.9525, -26.7669) -> (-95.2693, -14.5236) projected
  arc A12 (-94.6777, -12.8943) -> (-95.2693, -14.5236) centre (-94.5046, -13.8792) ccw projected
  arc A13 (-97.1203, -16.9825) -> (-98.885, -17.6269) centre (-97.885, -17.6269) ccw projected
  line L3 (-97.1203, -16.9825) -> (-87.2466, -28.7001) projected
  arc A14 (-87.3669, -30.1091) -> (-87.2466, -28.7001) centre (-88.0113, -29.3444) ccw projected
  line L4 (-87.3669, -30.1091) -> (-94.615, -36.2167) projected
  arc A15 (-96.2374, -35.6607) -> (-94.615, -36.2167) centre (-95.2594, -35.452) ccw projected
  arc A16 (-96.2374, -35.6607) -> (-98.7086, -29.9236) centre (-111.885, -39) ccw projected
  arc A17 (-98.885, -29.3564) -> (-98.7086, -29.9236) centre (-97.885, -29.3564) ccw projected
  line L5 (-98.885, -29.3564) -> (-98.885, -17.6269) projected
  line L6 (-97.8265, -46.769) -> (-61.9457, -16.5342) projected
  arc A18 (-60.3014, -17.2989) -> (-61.9457, -16.5342) centre (-61.3014, -17.2989) ccw projected
  line L7 (-60.3014, -17.2989) -> (-60.3014, -82.75) projected
  arc A19 (-60.3014, -82.75) -> (-57.9314, -88) centre (-53.3014, -82.75) ccw projected
  arc A20 (-58.5929, -89.75) -> (-57.9314, -88) centre (-58.5929, -88.75) ccw projected
  line L8 (-58.5929, -89.75) -> (-60.1853, -89.75) projected
  arc A21 (-61.1499, -89.0136) -> (-60.1853, -89.75) centre (-60.1853, -88.75) ccw projected
  arc A22 (-61.1499, -89.0136) -> (-71.5218, -75.0244) centre (-84.3014, -95.339) ccw projected
  line L9 (-71.5218, -75.0244) -> (-103.9807, -54.6052) projected
  arc A23 (-103.9445, -52.8906) -> (-103.9807, -54.6052) centre (-103.4483, -53.7587) ccw projected
  arc A24 (-103.9445, -52.8906) -> (-98.047, -47.0317) centre (-111.885, -39) ccw projected
  arc A25 (-97.8265, -46.769) -> (-98.047, -47.0317) centre (-97.1821, -47.5337) ccw projected
  circle A26 centre (-47.8869, -88.25) radius 1.5 projected
  arc A27 (-46.177, -92.4125) -> (-47.885, -83.75) centre (-47.8869, -88.25) ccw projected
  line L10 (-47.885, -83.75) -> (-53.3014, -83.75) projected
  arc A28 (-54.3014, -82.75) -> (-53.3014, -83.75) centre (-53.3014, -82.75) ccw projected
  line L11 (-54.3014, -82.75) -> (-54.3014, -10.5578) projected
  arc A29 (-53.9457, -9.7931) -> (-54.3014, -10.5578) centre (-53.3014, -10.5578) ccw projected
  line L12 (-53.9457, -9.7931) -> (-49.4443, -6) projected
  line L13 (-49.4443, -6) -> (-49.4443, -3) projected
  line L14 (-49.4443, -3) -> (-52.4443, -3) projected
  arc A30 (-54.4443, -3) -> (-52.4443, -3) centre (-53.4443, -3) ccw projected
  line L15 (-54.4443, -3) -> (-57.4443, -3) projected
  line L16 (-57.4443, -3) -> (-57.4443, -6) projected
  arc A31 (-59.4443, -6) -> (-57.4443, -6) centre (-58.4443, -6) ccw projected
  line L17 (-59.4443, -6) -> (-64.4443, -6) projected
  arc A32 (-66.4443, -6) -> (-64.4443, -6) centre (-65.4443, -6) ccw projected
  line L18 (-66.4443, -6) -> (-66.4443, -3) projected
  line L19 (-66.4443, -3) -> (-69.4443, -3) projected
  arc A33 (-71.4443, -3) -> (-69.4443, -3) centre (-70.4443, -3) ccw projected
  line L20 (-71.4443, -3) -> (-82.8897, -3) projected
  arc A34 (-84.8897, -3) -> (-82.8897, -3) centre (-83.8897, -3) ccw projected
  line L21 (-84.8897, -3) -> (-87.8897, -3) projected
  line L22 (-87.8897, -3) -> (-87.8897, -6) projected
  arc A35 (-89.8897, -6) -> (-87.8897, -6) centre (-88.8897, -6) ccw projected
  line L23 (-89.8897, -6) -> (-94.8897, -6) projected
  arc A36 (-96.8897, -6) -> (-94.8897, -6) centre (-95.8897, -6) ccw projected
  line L24 (-96.8897, -6) -> (-96.8897, -3) projected
  line L25 (-96.8897, -3) -> (-99.8897, -3) projected
  arc A37 (-101.8897, -3) -> (-99.8897, -3) centre (-100.8897, -3) ccw projected
  line L26 (-101.8897, -3) -> (-104.885, -3) projected
  line L27 (-104.885, -3) -> (-104.885, -31.8586) projected
  arc A38 (-119.127, -45.896) -> (-104.885, -31.8586) centre (-111.885, -39) ccw projected
  line L28 (-119.127, -45.896) -> (-127.6513, -45.7727) projected
  line L29 (-127.6513, -45.7727) -> (-121.0577, -50.8686) projected
  arc A39 (-121.0577, -50.8686) -> (-119.8722, -51.6966) centre (-111.885, -39) ccw projected
  line L30 (-119.8722, -51.6966) -> (-74.7167, -80.1031) projected
  arc A40 (-66.3014, -95.339) -> (-74.7167, -80.1031) centre (-84.3014, -95.339) ccw projected
  line L31 (-66.3014, -95.339) -> (-66.3014, -95.75) projected
  line L32 (-66.3014, -95.75) -> (-54.3014, -95.75) projected
  line L33 (-54.3014, -95.75) -> (-46.177, -92.4125) projected
  line L34 (-57.1634, -53.7587) -> (-121.3386, -53.7587) construction
  line L35 (-57.1634, -51.2587) -> (-121.3386, -51.2587)
  line L36 (-121.3386, -56.2587) -> (-57.1634, -56.2587)
  arc A41 (-57.1634, -56.2587) -> (-57.1634, -51.2587) centre (-57.1634, -53.7587) ccw
  arc A42 (-121.3386, -51.2587) -> (-121.3386, -56.2587) centre (-121.3386, -53.7587) ccw
  line L37 (-53.3014, -82.75) -> (-84.3014, -95.339) construction
  line L38 (-53.8657, -81.3602) -> (-84.8657, -93.9493)
  line L39 (-83.737, -96.7288) -> (-52.737, -84.1398)
  arc A43 (-52.737, -84.1398) -> (-53.8657, -81.3602) centre (-53.3014, -82.75) ccw
  arc A44 (-84.8657, -93.9493) -> (-83.737, -96.7288) centre (-84.3014, -95.339) ccw
  point P0 (0, 0)
  point P1 (-89.251, -53.7587)
  point P2 (-68.8014, -89.0445)
  dimension "d176" = 5
  dimension "d177" = 3
  constraints: 16 end point, 8 point on circle, 8 tangent, 4 centre point, 2 midpoint, 2 parallel, 1 horizontal, 1 point on line
  measures "d176" diameter of A42
  measures "d177" diameter of A44
sketch "スケッチ21" plane through (0, 0, -5) normal (0, 0, -1) x (-1, 0, 0)
  arc A0 (-94.6777, -12.8943) -> (-92.8272, -12.2945) centre (-95.8897, -6) ccw projected
  arc A1 (-91.9522, -12.2945) -> (-92.8272, -12.2945) centre (-92.3897, -13.1937) ccw projected
  arc A2 (-91.9522, -12.2945) -> (-83.3484, -10.2772) centre (-88.8897, -6) ccw projected
  arc A3 (-82.7234, -9.9022) -> (-83.3484, -10.2772) centre (-82.5568, -10.8882) ccw projected
  arc A4 (-82.7234, -9.9022) -> (-80.5008, -9.125) centre (-83.8897, -3) ccw projected
  arc A5 (-80.0167, -9) -> (-80.5008, -9.125) centre (-80.0167, -10) ccw projected
  line L0 (-80.0167, -9) -> (-74.3173, -9) projected
  arc A6 (-73.8332, -9.125) -> (-74.3173, -9) centre (-74.3173, -10) ccw projected
  arc A7 (-73.8332, -9.125) -> (-71.6106, -9.9022) centre (-70.4443, -3) ccw projected
  arc A8 (-70.9856, -10.2772) -> (-71.6106, -9.9022) centre (-71.7772, -10.8882) ccw projected
  arc A9 (-70.9856, -10.2772) -> (-68.4513, -12.3212) centre (-65.4443, -6) ccw projected
  arc A10 (-68.2365, -13.989) -> (-68.4513, -12.3212) centre (-68.8809, -13.2243) ccw projected
  line L1 (-68.2365, -13.989) -> (-83.5434, -26.8873) projected
  arc A11 (-84.9525, -26.7669) -> (-83.5434, -26.8873) centre (-84.1878, -26.1225) ccw projected
  line L2 (-84.9525, -26.7669) -> (-95.2693, -14.5236) projected
  arc A12 (-94.6777, -12.8943) -> (-95.2693, -14.5236) centre (-94.5046, -13.8792) ccw projected
  arc A13 (-97.1203, -16.9825) -> (-98.885, -17.6269) centre (-97.885, -17.6269) ccw projected
  line L3 (-97.1203, -16.9825) -> (-87.2466, -28.7001) projected
  arc A14 (-87.3669, -30.1091) -> (-87.2466, -28.7001) centre (-88.0113, -29.3444) ccw projected
  line L4 (-87.3669, -30.1091) -> (-94.615, -36.2167) projected
  arc A15 (-96.2374, -35.6607) -> (-94.615, -36.2167) centre (-95.2594, -35.452) ccw projected
  arc A16 (-96.2374, -35.6607) -> (-98.7086, -29.9236) centre (-111.885, -39) ccw projected
  arc A17 (-98.885, -29.3564) -> (-98.7086, -29.9236) centre (-97.885, -29.3564) ccw projected
  line L5 (-98.885, -29.3564) -> (-98.885, -17.6269) projected
  line L6 (-97.8265, -46.769) -> (-61.9457, -16.5342) projected
  arc A18 (-60.3014, -17.2989) -> (-61.9457, -16.5342) centre (-61.3014, -17.2989) ccw projected
  line L7 (-60.3014, -17.2989) -> (-60.3014, -82.75) projected
  arc A19 (-60.3014, -82.75) -> (-57.9314, -88) centre (-53.3014, -82.75) ccw projected
  arc A20 (-58.5929, -89.75) -> (-57.9314, -88) centre (-58.5929, -88.75) ccw projected
  line L8 (-58.5929, -89.75) -> (-60.1853, -89.75) projected
  arc A21 (-61.1499, -89.0136) -> (-60.1853, -89.75) centre (-60.1853, -88.75) ccw projected
  arc A22 (-61.1499, -89.0136) -> (-71.5218, -75.0244) centre (-84.3014, -95.339) ccw projected
  line L9 (-71.5218, -75.0244) -> (-103.9807, -54.6052) projected
  arc A23 (-103.9445, -52.8906) -> (-103.9807, -54.6052) centre (-103.4483, -53.7587) ccw projected
  arc A24 (-103.9445, -52.8906) -> (-98.047, -47.0317) centre (-111.885, -39) ccw projected
  arc A25 (-97.8265, -46.769) -> (-98.047, -47.0317) centre (-97.1821, -47.5337) ccw projected
  circle A26 centre (-47.8869, -88.25) radius 1.5 projected
  arc A27 (-46.177, -92.4125) -> (-47.885, -83.75) centre (-47.8869, -88.25) ccw projected
  line L10 (-47.885, -83.75) -> (-53.3014, -83.75) projected
  arc A28 (-54.3014, -82.75) -> (-53.3014, -83.75) centre (-53.3014, -82.75) ccw projected
  line L11 (-54.3014, -82.75) -> (-54.3014, -10.5578) projected
  arc A29 (-53.9457, -9.7931) -> (-54.3014, -10.5578) centre (-53.3014, -10.5578) ccw projected
  line L12 (-53.9457, -9.7931) -> (-49.4443, -6) projected
  line L13 (-49.4443, -6) -> (-49.4443, -3) projected
  line L14 (-49.4443, -3) -> (-52.4443, -3) projected
  arc A30 (-54.4443, -3) -> (-52.4443, -3) centre (-53.4443, -3) ccw projected
  line L15 (-54.4443, -3) -> (-57.4443, -3) projected
  line L16 (-57.4443, -3) -> (-57.4443, -6) projected
  arc A31 (-59.4443, -6) -> (-57.4443, -6) centre (-58.4443, -6) ccw projected
  line L17 (-59.4443, -6) -> (-64.4443, -6) projected
  arc A32 (-66.4443, -6) -> (-64.4443, -6) centre (-65.4443, -6) ccw projected
  line L18 (-66.4443, -6) -> (-66.4443, -3) projected
  line L19 (-66.4443, -3) -> (-69.4443, -3) projected
  arc A33 (-71.4443, -3) -> (-69.4443, -3) centre (-70.4443, -3) ccw projected
  line L20 (-71.4443, -3) -> (-82.8897, -3) projected
  arc A34 (-84.8897, -3) -> (-82.8897, -3) centre (-83.8897, -3) ccw projected
  line L21 (-84.8897, -3) -> (-87.8897, -3) projected
  line L22 (-87.8897, -3) -> (-87.8897, -6) projected
  arc A35 (-89.8897, -6) -> (-87.8897, -6) centre (-88.8897, -6) ccw projected
  line L23 (-89.8897, -6) -> (-94.8897, -6) projected
  arc A36 (-96.8897, -6) -> (-94.8897, -6) centre (-95.8897, -6) ccw projected
  line L24 (-96.8897, -6) -> (-96.8897, -3) projected
  line L25 (-96.8897, -3) -> (-99.8897, -3) projected
  arc A37 (-101.8897, -3) -> (-99.8897, -3) centre (-100.8897, -3) ccw projected
  line L26 (-101.8897, -3) -> (-104.885, -3) projected
  line L27 (-104.885, -3) -> (-104.885, -31.8586) projected
  arc A38 (-119.127, -45.896) -> (-104.885, -31.8586) centre (-111.885, -39) ccw projected
  line L28 (-119.127, -45.896) -> (-127.6513, -45.7727) projected
  line L29 (-127.6513, -45.7727) -> (-121.0577, -50.8686) projected
  arc A39 (-121.0577, -50.8686) -> (-119.8722, -51.6966) centre (-111.885, -39) ccw projected
  line L30 (-119.8722, -51.6966) -> (-74.7167, -80.1031) projected
  arc A40 (-66.3014, -95.339) -> (-74.7167, -80.1031) centre (-84.3014, -95.339) ccw projected
  line L31 (-66.3014, -95.339) -> (-66.3014, -95.75) projected
  line L32 (-66.3014, -95.75) -> (-54.3014, -95.75) projected
  line L33 (-54.3014, -95.75) -> (-46.177, -92.4125) projected
  line L34 (-72.5868, -76.7173) -> (-117.7423, -48.3109)
  arc A41 (-118.6116, -47.7036) -> (-117.7423, -48.3109) centre (-111.885, -39) ccw
  line L35 (-118.6116, -47.7036) -> (-126.6327, -41.5046)
  line L36 (-100.3297, -30.1495) -> (-100.3297, -9.3388)
  arc A42 (-100.3297, -9.3388) -> (-92.71, -10.5553) centre (-95.8897, -6) ccw
  line L37 (-92.71, -10.5553) -> (-92.0694, -10.5553)
  arc A43 (-92.0694, -10.5553) -> (-83.3344, -6) centre (-88.8897, -6) ccw
  line L38 (-83.3344, -6) -> (-83.3344, 2.5275)
  arc A44 (-83.3344, 2.5275) -> (-80.71, -7.5553) centre (-83.8897, -3) ccw
  line L39 (-80.71, -7.5553) -> (-73.6241, -7.5553)
  arc A45 (-73.6241, -7.5553) -> (-70.9997, 2.5275) centre (-70.4443, -3) ccw
  line L40 (-70.9997, 2.5275) -> (-70.9997, -6)
  arc A46 (-70.9997, -6) -> (-62.2646, -10.5553) centre (-65.4443, -6) ccw
  line L41 (-62.2646, -10.5553) -> (-61.6241, -10.5553)
  line L42 (-58.3014, -11.54) -> (-58.3014, -82.75)
  arc A47 (-58.3014, -82.75) -> (-53.3014, -87.75) centre (-53.3014, -82.75) ccw
  line L43 (-53.3014, -87.75) -> (-45.354, -87.75)
  line L44 (-45.354, -87.75) -> (-55.091, -91.75)
  line L45 (-55.091, -91.75) -> (-62.5961, -91.75)
  arc A48 (-62.5961, -91.75) -> (-72.5868, -76.7173) centre (-84.3014, -95.339) ccw
  circle A49 centre (-47.8869, -88.25) radius 5.5
  line L46 (-61.9457, -16.5342) -> (-58.3014, -13.4633)
  circle A50 centre (-111.885, -39) radius 1.5 projected
  arc A51 (-103.9445, -52.8906) -> (-103.9807, -54.6052) centre (-103.4483, -53.7587) ccw projected
  circle A52 centre (-111.885, -39) radius 16
  line L47 (-97.8265, -46.769) -> (-61.9457, -16.5342) projected
  point P0 (0, 0)
  point P1 (-52.7633, -90.7938)
  point P2 (-53.3641, -87.7496)
  point P3 (-107.9076, -54.4977)
  dimension "d178" = 4
  dimension "d179" = 4
  dimension "d180" = 4
  constraints: 26 end point, 16 point on circle, 9 centre point, 1 coincident, 1 collinear, 1 point on line, 20 other
  measures "d178" distance between parallel lines of L34 L30
  measures "d179" distance between parallel lines of L11 L42
  measures "d180" radial gap between concentric circles of A26 A49
extrude "押し出し23" cut sketch "スケッチ21" against normal blind 4 contours A23 L9 A22 A21 L8 A20 A19 L7 A18 L46 L42 A47 A49 L44 L45 A48 L34 A52
fillet "フィレット5" radius 1 6 edges at (53.3641, -87.7496, -3) (52.7633, -90.7938, -3) (55.091, -91.75, -3) (62.5961, -91.75, -3) (107.9076, -54.4977, -3) (58.3014, -13.4633, -3)
sketch "スケッチ22" plane through (0, 0, -5) normal (0, 0, -1) x (-1, 0, 0)
  arc A0 (-105.9445, -53.8563) -> (-98.047, -47.0317) centre (-111.885, -39) ccw projected
  arc A1 (-97.8265, -46.769) -> (-98.047, -47.0317) centre (-97.1821, -47.5337) ccw projected
  line L0 (-97.8265, -46.769) -> (-59.9457, -14.8489) projected
  arc A2 (-58.3014, -15.6137) -> (-59.9457, -14.8489) centre (-59.3014, -15.6137) ccw projected
  line L1 (-58.3014, -15.6137) -> (-58.3014, -82.75) projected
  arc A3 (-58.3014, -82.75) -> (-54.1956, -87.6694) centre (-53.3014, -82.75) ccw projected
  arc A4 (-53.3763, -88.5912) -> (-54.1956, -87.6694) centre (-54.3744, -88.6533) ccw projected
  arc A5 (-53.3763, -88.5912) -> (-53.1201, -89.9424) centre (-47.8869, -88.25) ccw projected
  arc A6 (-53.6916, -91.1751) -> (-53.1201, -89.9424) centre (-54.0715, -90.2501) ccw projected
  line L2 (-53.6916, -91.1751) -> (-54.9084, -91.675) projected
  arc A7 (-55.2884, -91.75) -> (-54.9084, -91.675) centre (-55.2884, -90.75) ccw projected
  line L3 (-55.2884, -91.75) -> (-61.7638, -91.75) projected
  arc A8 (-62.7437, -90.9495) -> (-61.7638, -91.75) centre (-61.7638, -90.75) ccw projected
  arc A9 (-62.7437, -90.9495) -> (-72.5868, -76.7173) centre (-84.3014, -95.339) ccw projected
  line L4 (-72.5868, -76.7173) -> (-106.1057, -55.6313) projected
  arc A10 (-105.9445, -53.8563) -> (-106.1057, -55.6313) centre (-105.5732, -54.7848) ccw projected
  arc A11 (-94.6777, -12.8943) -> (-92.8272, -12.2945) centre (-95.8897, -6) ccw projected
  arc A12 (-91.9522, -12.2945) -> (-92.8272, -12.2945) centre (-92.3897, -13.1937) ccw projected
  arc A13 (-91.9522, -12.2945) -> (-83.3484, -10.2772) centre (-88.8897, -6) ccw projected
  arc A14 (-82.7234, -9.9022) -> (-83.3484, -10.2772) centre (-82.5568, -10.8882) ccw projected
  arc A15 (-82.7234, -9.9022) -> (-80.5008, -9.125) centre (-83.8897, -3) ccw projected
  arc A16 (-80.0167, -9) -> (-80.5008, -9.125) centre (-80.0167, -10) ccw projected
  line L5 (-80.0167, -9) -> (-74.3173, -9) projected
  arc A17 (-73.8332, -9.125) -> (-74.3173, -9) centre (-74.3173, -10) ccw projected
  arc A18 (-73.8332, -9.125) -> (-71.6106, -9.9022) centre (-70.4443, -3) ccw projected
  arc A19 (-70.9856, -10.2772) -> (-71.6106, -9.9022) centre (-71.7772, -10.8882) ccw projected
  arc A20 (-70.9856, -10.2772) -> (-68.4513, -12.3212) centre (-65.4443, -6) ccw projected
  arc A21 (-68.2365, -13.989) -> (-68.4513, -12.3212) centre (-68.8809, -13.2243) ccw projected
  line L6 (-68.2365, -13.989) -> (-83.5434, -26.8873) projected
  arc A22 (-84.9525, -26.7669) -> (-83.5434, -26.8873) centre (-84.1878, -26.1225) ccw projected
  line L7 (-84.9525, -26.7669) -> (-95.2693, -14.5236) projected
  arc A23 (-94.6777, -12.8943) -> (-95.2693, -14.5236) centre (-94.5046, -13.8792) ccw projected
  arc A24 (-97.1203, -16.9825) -> (-98.885, -17.6269) centre (-97.885, -17.6269) ccw projected
  line L8 (-97.1203, -16.9825) -> (-87.2466, -28.7001) projected
  arc A25 (-87.3669, -30.1091) -> (-87.2466, -28.7001) centre (-88.0113, -29.3444) ccw projected
  line L9 (-87.3669, -30.1091) -> (-94.615, -36.2167) projected
  arc A26 (-96.2374, -35.6607) -> (-94.615, -36.2167) centre (-95.2594, -35.452) ccw projected
  arc A27 (-96.2374, -35.6607) -> (-98.7086, -29.9236) centre (-111.885, -39) ccw projected
  arc A28 (-98.885, -29.3564) -> (-98.7086, -29.9236) centre (-97.885, -29.3564) ccw projected
  line L10 (-98.885, -29.3564) -> (-98.885, -17.6269) projected
  circle A29 centre (-47.8869, -88.25) radius 1.5 projected
  arc A30 (-46.177, -92.4125) -> (-47.885, -83.75) centre (-47.8869, -88.25) ccw projected
  line L11 (-47.885, -83.75) -> (-53.3014, -83.75) projected
  arc A31 (-54.3014, -82.75) -> (-53.3014, -83.75) centre (-53.3014, -82.75) ccw projected
  line L12 (-54.3014, -82.75) -> (-54.3014, -10.5578) projected
  arc A32 (-53.9457, -9.7931) -> (-54.3014, -10.5578) centre (-53.3014, -10.5578) ccw projected
  line L13 (-53.9457, -9.7931) -> (-49.4443, -6) projected
  line L14 (-49.4443, -6) -> (-49.4443, -3) projected
  line L15 (-49.4443, -3) -> (-52.4443, -3) projected
  arc A33 (-54.4443, -3) -> (-52.4443, -3) centre (-53.4443, -3) ccw projected
  line L16 (-54.4443, -3) -> (-57.4443, -3) projected
  line L17 (-57.4443, -3) -> (-57.4443, -6) projected
  arc A34 (-59.4443, -6) -> (-57.4443, -6) centre (-58.4443, -6) ccw projected
  line L18 (-59.4443, -6) -> (-64.4443, -6) projected
  arc A35 (-66.4443, -6) -> (-64.4443, -6) centre (-65.4443, -6) ccw projected
  line L19 (-66.4443, -6) -> (-66.4443, -3) projected
  line L20 (-66.4443, -3) -> (-69.4443, -3) projected
  arc A36 (-71.4443, -3) -> (-69.4443, -3) centre (-70.4443, -3) ccw projected
  line L21 (-71.4443, -3) -> (-82.8897, -3) projected
  arc A37 (-84.8897, -3) -> (-82.8897, -3) centre (-83.8897, -3) ccw projected
  line L22 (-84.8897, -3) -> (-87.8897, -3) projected
  line L23 (-87.8897, -3) -> (-87.8897, -6) projected
  arc A38 (-89.8897, -6) -> (-87.8897, -6) centre (-88.8897, -6) ccw projected
  line L24 (-89.8897, -6) -> (-94.8897, -6) projected
  arc A39 (-96.8897, -6) -> (-94.8897, -6) centre (-95.8897, -6) ccw projected
  line L25 (-96.8897, -6) -> (-96.8897, -3) projected
  line L26 (-96.8897, -3) -> (-99.8897, -3) projected
  arc A40 (-101.8897, -3) -> (-99.8897, -3) centre (-100.8897, -3) ccw projected
  line L27 (-101.8897, -3) -> (-104.885, -3) projected
  line L28 (-104.885, -3) -> (-104.885, -31.8586) projected
  arc A41 (-119.127, -45.896) -> (-104.885, -31.8586) centre (-111.885, -39) ccw projected
  line L29 (-119.127, -45.896) -> (-127.6513, -45.7727) projected
  line L30 (-127.6513, -45.7727) -> (-121.0577, -50.8686) projected
  arc A42 (-121.0577, -50.8686) -> (-119.8722, -51.6966) centre (-111.885, -39) ccw projected
  line L31 (-119.8722, -51.6966) -> (-74.7167, -80.1031) projected
  arc A43 (-66.3014, -95.339) -> (-74.7167, -80.1031) centre (-84.3014, -95.339) ccw projected
  line L32 (-66.3014, -95.339) -> (-66.3014, -95.75) projected
  line L33 (-66.3014, -95.75) -> (-54.3014, -95.75) projected
  line L34 (-54.3014, -95.75) -> (-46.177, -92.4125) projected
  line L35 (-53.3014, -82.75) -> (-84.3014, -95.339) construction
  line L36 (-54.0539, -80.897) -> (-85.0539, -93.486)
  line L37 (-83.5488, -97.1921) -> (-52.5488, -84.603)
  arc A44 (-52.5488, -84.603) -> (-54.0539, -80.897) centre (-53.3014, -82.75) ccw
  arc A45 (-85.0539, -93.486) -> (-83.5488, -97.1921) centre (-84.3014, -95.339) ccw
  line L38 (-35.2454, -54.7848) -> (-127.8382, -54.7848) construction
  line L39 (-35.2454, -52.2848) -> (-127.8382, -52.2848)
  line L40 (-127.8382, -57.2848) -> (-35.2454, -57.2848)
  arc A46 (-35.2454, -57.2848) -> (-35.2454, -52.2848) centre (-35.2454, -54.7848) ccw
  arc A47 (-127.8382, -52.2848) -> (-127.8382, -57.2848) centre (-127.8382, -54.7848) ccw
  point P0 (0, 0)
  point P1 (-68.8014, -89.0445)
  point P2 (-81.5418, -54.7848)
  point P3 (-103.4771, -57.2848)
  point P4 (-58.3014, -57.2848)
  point P5 (-58.3014, -52.2848)
  point P6 (-102.968, -52.2848)
  point P7 (-63.2499, -88.9487)
  point P8 (-56.7947, -86.3273)
  point P9 (-58.3014, -82.6219)
  point P10 (-64.7549, -85.2427)
  dimension "d184" = 4
  dimension "d185" = 5
  constraints: 16 end point, 8 point on circle, 8 tangent, 4 centre point, 2 midpoint, 2 parallel, 1 horizontal, 1 point on line
  measures "d184" diameter of A45
  measures "d185" diameter of A47
extrude "押し出し24" add sketch "スケッチ22" against normal blind 5 contours A0 L39 L1 L40 L4 A10 | L1 A3 L37 A9 L36
fillet "フィレット6" radius 1 8 edges at (58.3014, -82.6219, -3) (56.7947, -86.3273, -3) (63.2499, -88.9487, -3) (64.7549, -85.2427, -3) (103.4771, -57.2848, -3) (102.968, -52.2848, -3) (58.3014, -52.2848, -3) (58.3014, -57.2848, -3)